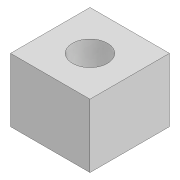
# Autodesk Inventor part: Shaft tool for motor
Saved by Autodesk Inventor 2020 (Build 240168000, 168)
## iProperties
Created: 2020-03-06
Part Number: Shaft tool for motor
Material: Generic
Document SubType Name: Modeling
Designer: ball
Density: 1 g/cm^3
Appearance: Default
Author: ball
Autodesk Inventor part; units mm, degrees
ref_plane "YZ Plane" through (0, 0, 0) normal (1, 0, 0) x (0, 1, 0)
ref_plane "XZ Plane" through (0, 0, 0) normal (0, 1, 0) x (-1, 0, 0)
ref_plane "XY Plane" through (0, 0, 0) normal (0, 0, 1) x (1, 0, 0)
sketch "Sketch1" plane through (0, 0, 0) normal (0, 1, 0) x (-1, 0, 0)
  line L0 (9.525, 9.525) -> (-9.525, 9.525)
  line L1 (-9.525, 9.525) -> (-9.525, -9.525)
  line L2 (-9.525, -9.525) -> (9.525, -9.525)
  line L3 (9.525, -9.525) -> (9.525, 9.525)
  line L4 (9.525, 9.525) -> (-9.525, -9.525) construction
  line L5 (-9.525, 9.525) -> (9.525, -9.525) construction
  circle A0 centre (0, 0) radius 4 construction
  dimension "d0" = 19.05
  dimension "d1" = 19.05
  dimension "d2" = 8
  constraints: 12 end point, 2 midpoint, 2 parallel, 1 centre point, 1 coincident, 1 horizontal, 1 perpendicular
  measures "d0" distance of L2.end L1.end
  measures "d1" distance of L1.end L0.end
  measures "d2" diameter of A0
extrude "Extrusion1" add sketch "Sketch1" along normal blind 15.24
sketch "Sketch2" plane through (0, 15.24, 0) normal (0, 1, 0) x (1, 0, 0)
  circle A0 centre (0, 0) radius 4.2
  dimension "d5" = 8.4
  constraints: 1 centre point, 1 coincident
  measures "d5" diameter of A0
extrude "Extrusion2" cut sketch "Sketch2" against normal blind 12.2428
body "Solid1"
